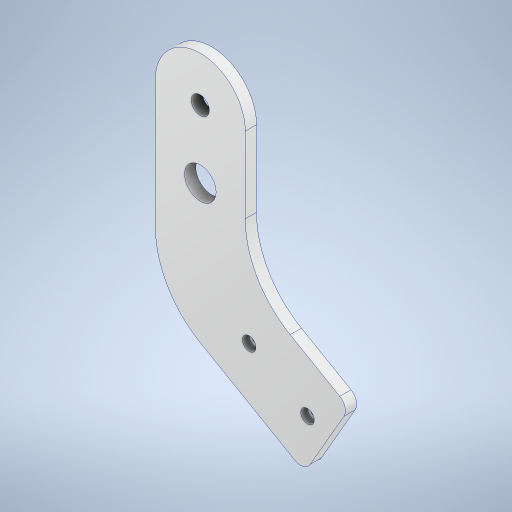
# Autodesk Inventor part: BR_parts_06(1)
Saved by Autodesk Inventor 2024.3 (Build 283343000, 343)
## iProperties
Created: 2024-10-20
Part Number: BR_parts_06(1)
Material: アルミニウム 6061
Document SubType Name: Modeling
Designer: 佐藤智貴
Density: 2.7 g/cm^3
Appearance: アルミニウム - フラット
Mass: 47.4329 g
Surface Area: 130.032 cm^2
Volume: 17.5677 cm^3
Author: 佐藤智貴
Autodesk Inventor part; units mm, degrees
ref_plane "YZ Plane" through (0, 0, 0) normal (1, 0, 0) x (0, 1, 0)
ref_plane "XZ Plane" through (0, 0, 0) normal (0, 1, 0) x (-1, 0, 0)
ref_plane "XY Plane" through (0, 0, 0) normal (0, 0, 1) x (1, 0, 0)
sketch "スケッチ1" plane through (0, 0, 0) normal (0, 0, 1) x (1, 0, 0)
  line L0 (0, 0) -> (40, 0)
  line L1 (40, 0) -> (40, 318)
  line L2 (40, 318) -> (0, 318)
  line L3 (0, 318) -> (0, 0)
  line L4 (0, 218) -> (112.7627, 152.8964)
  line L5 (112.7627, 152.8964) -> (132.7627, 187.5375)
  line L6 (132.7627, 187.5375) -> (40, 241.094)
  point P0 (40, 218)
  point P1 (40, 194.906)
  point P2 (20, 318)
  point P3 (122.7627, 170.2169)
  point P4 (20, 258)
  dimension "d0" = 40
  dimension "d1" = 318
  dimension "d69" = 40
  dimension "d70" = 60
  dimension "d91" = 20
  dimension "d92" = 100
  dimension "d93" = 180
  dimension "d96" = 20
  dimension "d97" = 60
  constraints: 14 end point, 3 perpendicular, 3 point on line, 2 midpoint, 2 parallel, 1 horizontal
  measures "d0" distance of L1.end L2.end
  measures "d1" distance of L0.end L1.end
  measures "d69" distance of L4.end L5.end
  measures "d70" angle of L3 L4
  measures "d91" distance from line of L6 point (40, 218)
  measures "d92" distance from line of L2 L4.start
  measures "d93" distance of point (20, 318) point (122.763, 170.217)
  measures "d96" distance from line of L1 point (20, 258)
  measures "d97" distance from line of L2 point (20, 258)
extrude "押し出し1" add sketch "スケッチ1" along normal blind 19.6 contours L3 L2 L1 L4 | L1 L6 L5 L4
sketch "スケッチ6" plane through (0, 0, 19.6) normal (0, 0, 1) x (1, 0, 0)
  circle A0 centre (20, 268) radius 7
  line L0 (40, 318) -> (0, 318) projected
  line L1 (40, 241.094) -> (40, 318) projected
  circle A1 centre (20, 20) radius 1.2295
  circle A2 centre (20, 10) radius 1.2295
  line L2 (0, 0) -> (40, 0) projected
  circle A3 centre (20, 298) radius 4
  point P0 (20, 318)
  point P1 (40, 190.8114)
  point P2 (30, 0)
  dimension "d42" = 14
  dimension "d44" = 20
  dimension "d45" = 2.459
  dimension "d46" = 2.459
  dimension "d47" = 10
  dimension "d48" = 10
  dimension "d49" = 20
  dimension "d50" = 20
  dimension "d53" = 8
  dimension "d54" = 20
  dimension "d55" = 30
  dimension "d56" = 20
  constraints: 4 centre point, 1 midpoint
  measures "d42" diameter of A0
  measures "d44" distance from line of L1 A0.centre
  measures "d45" diameter of A1
  measures "d46" diameter of A2
  measures "d47" distance from line of L2 A2.centre
  measures "d48" distance of A2.centre A1.centre
  measures "d49" distance from line of L1 A2.centre
  measures "d50" distance from line of L1 A1.centre
  measures "d53" diameter of A3
  measures "d54" distance from line of L0 A3.centre
  measures "d55" distance of A3.centre A0.centre
  measures "d56" distance from line of L1 A3.centre
extrude "押し出し4" cut sketch "スケッチ6" against normal through all contours A0 | A3
sketch "スケッチ8" plane through (0, 0, 0) normal (-1, 0, 0) x (0, 0, 1)
  line L0 (0, 318) -> (19.6, 318) projected
  line L1 (5, 318) -> (14.6, 318)
  line L2 (14.6, 318) -> (14.6, 278)
  line L3 (14.6, 278) -> (5, 278)
  line L4 (5, 278) -> (5, 318)
  line L5 (0, 318) -> (0, 0) projected
  dimension "d57" = 5
  dimension "d58" = 9.6
  dimension "d59" = 40
  dimension "d98" = 19.6
  constraints: 8 end point, 2 parallel, 1 horizontal, 1 perpendicular, 1 point on line
  measures "d57" distance between parallel lines of L5 L4
  measures "d58" distance between parallel lines of L4 L2
  measures "d59" distance between parallel lines of L0 L3
  measures "d98" distance of L0.start L0.end
extrude "押し出し5" cut sketch "スケッチ8" against normal through all
fillet "フィレット1" radius 20 4 edges at (40, 318, 17.1) (40, 318, 2.5) (0, 318, 2.5) (0, 318, 17.1)
fillet "フィレット2" radius 40 2 edges at (0, 218, 9.8) (40, 241.094, 9.8)
sketch "スケッチ9" plane through (0, 0, 19.6) normal (0, 0, 1) x (1, 0, 0)
  line L0 (20, 206.453) -> (112.7627, 152.8964) projected
  line L1 (132.7627, 187.5375) -> (60, 229.547) projected
  line L2 (112.7627, 152.8964) -> (132.7627, 187.5375) projected
  line L3 (132.7627, 187.5375) -> (112.7627, 152.8964)
  line L4 (66.3813, 179.6747) -> (112.7627, 152.8964)
  line L5 (132.7627, 187.5375) -> (166.773, 167.9016)
  line L6 (115.1204, 126.9801) -> (133.5174, 158.8446)
  line L7 (141.7531, 173.1092) -> (128.7627, 180.6092)
  line L8 (112.7627, 152.8964) -> (20, 206.453)
  line L9 (132.7627, 187.5375) -> (60, 229.547)
  line L10 (115.1204, 126.9801) -> (125.7531, 145.3964)
  line L11 (133.5174, 158.8446) -> (145.7531, 180.0375)
  line L12 (116.7627, 159.8246) -> (129.7531, 152.3246)
  line L13 (66.3813, 179.6747) -> (129.7531, 152.3246)
  line L14 (66.3813, 179.6747) -> (86.3813, 214.3157)
  line L15 (86.3813, 214.3157) -> (141.7531, 173.1092)
  point P0 (0, 0)
  point P1 (254.4532, 80.329)
  point P2 (128.7627, 180.6092)
  point P3 (123.2579, 156.0746)
  point P4 (86.3813, 214.3157)
  point P5 (40, 194.906)
  point P6 (115.8875, 158.3088)
  point P7 (129.6379, 182.1251)
  dimension "d80" = 24
  dimension "d81" = 40
  dimension "d83" = 15
  dimension "d84" = 8
  dimension "d90" = 24
  constraints: 26 end point, 9 point on line, 6 perpendicular, 2 collinear, 2 midpoint, 1 parallel
  measures "d80" distance from line of point (254.453, 80.329) L7
  measures "d81" distance of L0.end L1.start
  measures "d83" distance between parallel lines of L2 L6
  measures "d84" distance between parallel lines of L5 L7
  measures "d90" distance from line of point (123.258, 156.075) L7
extrude "押し出し6" cut sketch "スケッチ9" against normal through all contours L13 L2 L0 | L1 L2 L15
sketch "スケッチ11" plane through (104.9897, 139.4332, 24) normal (0.8660254, -0.5, 0) x (0, 0, -1)
  line L0 (4.4, 21.7957) -> (4.4, 49.2964) projected
  line L1 (24, 21.7957) -> (24, 49.2964) projected
  line L2 (0, 24) -> (24, 24)
  line L3 (24, 24) -> (24, 0)
  line L4 (24, 0) -> (0, 0)
  line L5 (0, 0) -> (0, 24)
  line L6 (17, 17) -> (7, 17)
  line L7 (7, 17) -> (7, 7)
  line L8 (7, 7) -> (17, 7)
  line L9 (17, 7) -> (17, 17)
  line L10 (4.4, 35.546) -> (24, 35.546) projected
  circle A0 centre (14.2, 35.546) radius 5
  point P0 (24, -173.2475)
  point P1 (24, 24)
  point P2 (0, 15.546)
  point P3 (24, 15.546)
  dimension "d85" = 10
  dimension "d88" = 10
  constraints: 16 end point, 4 parallel, 2 perpendicular, 1 centre point, 1 horizontal, 1 midpoint, 4 other
  measures "d85" distance of L6.start L6.end
  measures "d88" diameter of A0
extrude "押し出し7" add sketch "スケッチ11" along normal blind 15 contours A0 L10 | L10 A0
fillet "フィレット4" radius 20 2 edges at (0, 278, 9.8) (40, 278, 9.8)
sketch "スケッチ12" plane through (0, 0, 19.6) normal (0, 0, 1) x (1, 0, 0)
  line L0 (0, 340.2847) -> (40, 340.2847)
  line L1 (40, 340.2847) -> (40, 181.2581)
  line L2 (40, 181.2581) -> (0, 181.2581)
  line L3 (0, 181.2581) -> (0, 340.2847)
  line L4 (40, 264.188) -> (40, 298) projected
  arc A0 (40, 298) -> (0, 298) centre (20, 298) ccw
  arc A1 (40, 264.188) -> (60, 229.547) centre (80, 264.188) ccw projected
  line L5 (60, 229.547) -> (40, 194.906)
  line L6 (20, 206.453) -> (66.3813, 179.6747) projected
  arc A2 (0, 241.094) -> (20, 206.453) centre (40, 241.094) ccw projected
  arc A3 (0, 241.094) -> (20, 206.453) centre (40, 241.094) ccw
  line L7 (20, 206.453) -> (40, 194.906)
  line L8 (86.3813, 214.3157) -> (60, 229.547) projected
  line L9 (60, 229.547) -> (86.3813, 214.3157)
  line L10 (86.3813, 214.3157) -> (66.3813, 179.6747)
  line L11 (40, 194.906) -> (66.3813, 179.6747)
  circle A4 centre (20, 298) radius 4
  circle A5 centre (20, 268) radius 7 projected
  circle A6 centre (20, 268) radius 4
  point P0 (0, 0)
  dimension "d99" = 40
  dimension "d100" = 40
  constraints: 18 end point, 4 centre point, 4 point on circle, 3 collinear, 3 point on line, 2 coincident, 2 parallel, 2 perpendicular, 2 tangent, 1 horizontal
  measures "d99" distance between parallel lines of L3 L4
  measures "d100" distance between parallel lines of L3 L1
extrude "押し出し8" add sketch "スケッチ12" along normal blind 5 contours A0 L1 L6 A2 L3 | A1 L5 L1 | L5 L8 L10 L6
sketch "スケッチ13" plane through (0, 0, 0) normal (0, 0, -1) x (-1, 0, 0)
  line L0 (-253.843, 397.4333) -> (123.9074, 397.4333)
  line L1 (123.9074, 397.4333) -> (123.9074, 95.9261)
  line L2 (123.9074, 95.9261) -> (-253.843, 95.9261)
  line L3 (-253.843, 95.9261) -> (-253.843, 397.4333)
  point P0 (0, 0)
  constraints: 8 end point, 2 parallel, 1 horizontal, 1 perpendicular
extrude "押し出し9" cut sketch "スケッチ13" against normal blind 19.6
sketch "スケッチ14" plane through (0, 0, 24.6) normal (0, 0, 1) x (1, 0, 0)
  line L0 (20, 206.453) -> (66.3813, 179.6747) projected
  line L1 (66.3813, 179.6747) -> (86.3813, 214.3157) projected
  line L2 (41.7403, 216.9952) -> (76.3813, 196.9952)
  point P0 (0, 0)
  point P1 (67.7211, 201.9952)
  dimension "d105" = 20
  dimension "d106" = 20
  dimension "d107" = 30
  dimension "d108" = 10
  constraints: 2 end point, 1 midpoint
  measures "d105" distance from line of L0 point (67.721, 201.995)
  measures "d106" distance from line of L0 L2.start
  measures "d107" distance of point (67.721, 201.995) L2.start
  measures "d108" distance from line of L1 point (67.721, 201.995)
hole "穴3" at (41.7403, 216.9952, 24.6) at (67.7211, 201.9952, 24.6) direction (0, 0, -1) diameter 3 end through all
fillet "フィレット5" radius 5 2 edges at (86.3813, 214.3157, 22.1) (66.3813, 179.6747, 22.1)
sketch "スケッチ15" plane through (0, 0, 24.6) normal (0, 0, 1) x (1, 0, 0)
  circle A0 centre (41.7403, 216.9952) radius 1.5 projected
  circle A1 centre (41.7403, 216.9952) radius 3
  circle A2 centre (67.7211, 201.9952) radius 1.5 projected
  circle A3 centre (67.7211, 201.9952) radius 3
  point P0 (0, 0)
  dimension "d117" = 6
  dimension "d118" = 6
  constraints: 2 centre point, 2 coincident
  measures "d117" diameter of A1
  measures "d118" diameter of A3
extrude "押し出し10" cut sketch "スケッチ15" against normal blind 3
equation "\"d45\" = d46"
equation "\"d48\" = d47"
equation "\"d50\" = d49"
equation "\"d106\" = d105"
